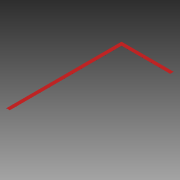
# Autodesk Inventor part: protected zone tape Red
Saved by Autodesk Inventor 2015 (Build 190159000, 159)
## iProperties
Created: 2015-04-21
Part Number: protected zone tape Red
Material: Generic
Document SubType Name: Modeling
Designer: David Tenney
Density: 1 g/cm^3
Appearance: Default
Author: David Tenney
Autodesk Inventor part; units mm, degrees
ref_plane "YZ Plane" through (0, 0, 0) normal (1, 0, 0) x (0, 1, 0)
ref_plane "XZ Plane" through (0, 0, 0) normal (0, 1, 0) x (-1, 0, 0)
ref_plane "XY Plane" through (0, 0, 0) normal (0, 0, 1) x (1, 0, 0)
sketch "Sketch1" plane through (2835.9464, 0.127, -1682.1632) normal (0, 1, 0) x (1, 0, 0)
  line L0 (0, -1676.4) -> (50.8001, -1676.4) projected
  line L1 (50.8001, -1676.4) -> (50.8001, -50.8) projected
  line L2 (50.8001, -50.8) -> (758.8544, -50.8) projected
  line L3 (758.8544, -50.8) -> (758.7571, 0) construction
  line L4 (758.7571, 0) -> (0, 0) projected
  line L5 (0, 0) -> (0, -1676.4) projected
  line L6 (758.8544, -50.8) -> (758.8544, 0)
  line L7 (758.8544, -50.8) -> (809.6544, -50.8) construction
  line L8 (758.8544, 0) -> (0, 0)
  line L9 (0, 0) -> (0, -1676.4)
  line L10 (0, -1676.4) -> (50.8001, -1676.4)
  line L11 (50.8001, -1676.4) -> (50.8001, -50.8)
  line L12 (50.8001, -50.8) -> (758.8544, -50.8)
  point P0 (-2835.9464, -1682.1632)
  dimension "d0" = 90
  dimension "d1" = 90
  dimension "d2" = 90
  constraints: 14 end point, 4 horizontal, 2 vertical, 1 perpendicular, 1 point on line
  measures "d0" angle of L7 L6
  measures "d1" angle of L10 L9
  measures "d2" angle of L11 L12
extrude "Extrusion1" add sketch "Sketch1" against normal blind 0.127
